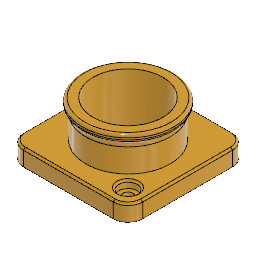
spool_axis v4 (Autodesk Fusion 360 design; units mm, degrees)
Autodesk Fusion 360 part; units mm, degrees
note: some values were not read from the file. Set by a fixed rule: which sketch regions a step uses.
sketch "Sketch1" plane through (0, 0, 0) normal (0, 0, 1) x (1, 0, 0)
  circle A0 centre (0, 0) radius 25
  circle A1 centre (0, 0) radius 23
  circle A2 centre (0, 0) radius 19
  circle A3 centre (22.6274, -22.6274) radius 5
  circle A4 centre (22.6274, -22.6274) radius 2.7
  circle A5 centre (-22.6274, 22.6274) radius 5
  circle A6 centre (-22.6274, 22.6274) radius 2.7
  line L0 (32.5, -32.5) -> (-32.5, -32.5)
  line L1 (-32.5, -32.5) -> (-32.5, 32.5)
  line L2 (-32.5, 32.5) -> (32.5, 32.5)
  line L3 (32.5, 32.5) -> (32.5, -32.5)
  line L4 (32.5, -32.5) -> (-32.5, 32.5) construction
  line L5 (-32.5, -32.5) -> (32.5, 32.5) construction
  dimension "d1" = 50
  dimension "d2" = 46
  dimension "d3" = 38
  dimension "d16" = 10
  dimension "d18" = 5.4
  dimension "d19" = 5.4
  dimension "d20" = 10
  dimension "d25" = 32
  dimension "d26" = 32
  dimension "d27" = 65
  constraint coincident A0.centre A1.centre
  constraint concentric A0 A1
  constraint concentric A1 A2
  constraint concentric A3 A4
  constraint concentric A5 A6
  constraint perpendicular L0 L1
  constraint parallel L0 L2
  constraint parallel L1 L3
  constraint horizontal L0
  constraint coincident L4 A0.centre
  constraint coincident L5 A0.centre
  constraint coincident A3.centre L4
  constraint coincident A5.centre L4
  measures "d1" diameter of A0
  measures "d2" diameter of A1
  measures "d3" diameter of A2
  measures "d16" diameter of A3
  measures "d18" diameter of A4
  measures "d19" diameter of A6
  measures "d20" diameter of A5
  measures "d25" distance of A0.centre A3.centre
  measures "d26" distance of A0.centre A5.centre
  measures "d27" distance of L0.start L2.end
extrude "Extrude1" add sketch "Sketch1" along normal blind 9 contours A0 | A1 | A3 | A5 | L0 L1 L2 L3
extrude "Extrude2" add sketch "Sketch1" along normal blind 20 from surface at 9 contours A1
extrude "Extrude3" add sketch "Sketch1" against normal blind 4 from surface at 29 contours A0
fillet "Fillet1" radius 1.5 2 edges at (-23.3082, 9.0404, 29) (-23.3082, 9.0404, 25)
fillet "Fillet2" radius 5 1 edges at (-21.4435, 8.3172, 25)
extrude "Extrude4" cut sketch "Sketch1" along normal up to surface (4 mm away) from surface at 5 contours A3 | A5
fillet "Fillet3" radius 8 4 edges at (-32.5, -32.5, 4.5) (32.5, -32.5, 4.5) (32.5, 32.5, 4.5) (-32.5, 32.5, 4.5)
chamfer "Chamfer1" distance 1 angle 45 10 edges at (-27.2891, 24.4355, 9) (17.9658, -20.8193, 9) (-30.1569, 30.1569, 9) (-32.5, 0, 9) (-30.1569, -30.1569, 9) (0, -32.5, 9) (30.1569, -30.1569, 9) (32.5, 0, 9) (30.1569, 30.1569, 9) (0, 32.5, 9)
equation "d2 = d1 - ( 2 * 2 ) * 1 mm"
equation "d3 = d2 - ( 2 * 4 ) * 1 mm"
equation "d19 = d18"
equation "d20 = d16"
equation "d26 = d25"
